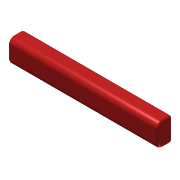
# Autodesk Inventor part: SideBumpers
Saved by Autodesk Inventor 2013 (Build 170138000, 138)
## iProperties
Created: 2013-05-20
Part Number: SideBumpers
Material: Generic
Document SubType Name: Modeling
Designer: Nemo
Density: 0.180591 g/cm^3
Mass: 1451.5 g
Surface Area: 3233.63 cm^2
Volume: 8037.49 cm^3
Author: Nemo
Autodesk Inventor part; units mm, degrees
ref_plane "YZ Plane" through (0, 0, 0) normal (1, 0, 0) x (0, 1, 0)
ref_plane "XZ Plane" through (0, 0, 0) normal (0, 1, 0) x (-1, 0, 0)
ref_plane "XY Plane" through (0, 0, 0) normal (0, 0, 1) x (1, 0, 0)
sketch "Sketch1" plane through (0, 0, 0) normal (0, 0, 1) x (1, 0, 0)
  line L0 (-403.86, 63.5) -> (403.86, 63.5)
  line L1 (403.86, 63.5) -> (403.86, -63.5)
  line L2 (403.86, -63.5) -> (-403.86, -63.5)
  line L3 (-403.86, -63.5) -> (-403.86, 63.5)
  point P0 (0, 0)
  point P1 (-403.86, 0)
  point P2 (0, 63.5)
  dimension "d0" = 807.72
  dimension "d1" = 127
  constraints: 8 end point, 2 midpoint, 2 parallel, 1 horizontal, 1 horizontal alignment, 1 perpendicular, 1 vertical alignment
  measures "d0" distance of L1.end L2.end
  measures "d1" distance of L0.end L1.end
extrude "Extrusion1" add sketch "Sketch1" along normal blind 19.05
sketch "Sketch2" plane through (0, 0, 0) normal (1, 0, 0) x (0, 1, 0)
  line L0 (63.5, 19.05) -> (63.5, 0) construction
  line L1 (63.5, 0) -> (-63.5, 0) construction
  line L2 (-63.5, 0) -> (-63.5, 19.05) construction
  line L3 (-63.5, 19.05) -> (63.5, 19.05) construction
  circle A0 centre (31.75, 50.8) radius 31.75
  circle A1 centre (-31.75, 50.8) radius 31.75
  point P0 (0, 0)
  dimension "d4" = 63.5
  dimension "d5" = 63.5
  constraints: 4 tangent, 2 centre point
  measures "d4" diameter of A0
  measures "d5" diameter of A1
extrude "Extrusion2" add sketch "Sketch2" along normal mid plane 807.72
sketch "Sketch4" plane through (403.86, -63.5, 0) normal (1, 0, 0) x (0, 0, -1)
  line L0 (-19.05, 127) -> (0, 127) projected
  line L1 (0, 127) -> (0, 0) projected
  line L2 (0, 0) -> (-19.05, 0) projected
  line L3 (-19.05, 0) -> (-19.05, 31.75) projected
  line L4 (-19.05, 31.75) -> (-19.05, 95.25) projected
  arc A0 (-50.8, 63.5) -> (-19.05, 95.25) centre (-50.8, 95.25) ccw projected
  arc A1 (-50.8, 63.5) -> (-19.05, 31.75) centre (-50.8, 31.75) ccw projected
  arc A2 (-19.05, 31.75) -> (-50.8, 63.5) centre (-50.8, 31.75) ccw projected
  arc A3 (-19.05, 95.25) -> (-50.8, 63.5) centre (-50.8, 95.25) ccw projected
  line L5 (-19.05, 95.25) -> (-19.05, 127) projected
  line L6 (-19.05, 127) -> (-50.8, 127)
  line L7 (-82.55, 95.25) -> (-82.55, 31.75)
  line L8 (-50.8, 0) -> (-19.05, 0)
  point P0 (0, 63.5)
  constraints: 6 end point, 4 point on circle, 3 perpendicular, 2 tangent
extrude "Extrusion4" add sketch "Sketch4" against normal blind 807.72 contours L5 A3 L6 | L4 A2 A0 | L3 L8 A1 | A1 L7 A3
fillet "Fillet1" radius 12.7 14 edges at (0, 63.5, 0) (403.86, 0, 0) (0, -63.5, 0) (-403.86, 0, 0) (403.86, -63.5, 25.4) (-403.86, -63.5, 25.4) (403.86, -54.2006, 73.2506) (403.86, 0, 82.55) (403.86, 54.2006, 73.2506) (403.86, 63.5, 25.4) (-403.86, -54.2006, 73.2506) (-403.86, 0, 82.55) (-403.86, 54.2006, 73.2506) (-403.86, 63.5, 25.4)
equation "\"d6\" = d0"
equation "\"d10\" = d0"
body "Solid1"
